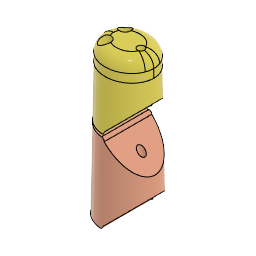
Thumb (Autodesk Fusion 360 design; units mm, degrees)
part number: 2025-12-08-00-09-45-361
part number: 2025-12-08-00-10-08-646
part number: 2025-12-08-00-15-25-462
Autodesk Fusion 360 part; units mm, degrees
sketch "Sketch1" plane through (0, 0, 0) normal (0, 0, 1) x (1, 0, 0) in component "Proximal phalanx"
  ellipse E0 centre (0, 0) end of major axis (0, -9) minor radius 10
  line L0 (0, 9) -> (0, -9) construction
  line L1 (-10, 0) -> (10, 0) construction
  dimension "d1" = 18
  dimension "d2" = 20
  constraint coincident E0 L0.start
  constraint coincident E0 L0.end
  constraint coincident E0 L1.start
  constraint coincident E0 L1.end
  constraint coincident E0.centre origin
  constraint vertical L0
  measures "d1" distance of E0
ref_plane "WorkPlane1" through (0, 0, 28) normal (0, 0, 1) x (1, 0, 0) in component "Proximal phalanx"
sketch "Sketch2" plane through (0, 0, 28) normal (0, 0, 1) x (1, 0, 0) in component "Proximal phalanx"
  ellipse E0 centre (0, 0) end of major axis (10, 0) minor radius 9
  spline S0 degree 3 poles (-9.5, 0) (-9.5, -2.2108) (-8.491, -4.4133) (-6.7366, -5.9923) (-5.0094, -7.5468) (-2.5777, -8.4723) (-0.1165, -8.4994) (2.3291, -8.5262) (4.7706, -7.6659) (6.5373, -6.1665) (8.3249, -4.6493) (9.4028, -2.5017) (9.4935, -0.3149) (9.5862, 1.9206) (8.6455, 4.1803) (6.9214, 5.8213) (5.2517, 7.4105) (2.8652, 8.3954) (0.4176, 8.4918) (-2.0105, 8.5874) (-4.4666, 7.8077) (-6.2824, 6.3751) (-8.121, 4.9244) (-9.2833, 2.8271) (-9.4715, 0.6572) (-9.4905, 0.4386) (-9.5, 0.2193) (-9.5, 0) knots -3.141593 -3.141593 -3.141593 -3.141593 -2.356194 -2.356194 -2.356194 -1.582994 -1.582994 -1.582994 -0.814704 -0.814704 -0.814704 -0.037301 -0.037301 -0.037301 0.757422 0.757422 0.757422 1.527054 1.527054 1.527054 2.290564 2.290564 2.290564 3.06369 3.06369 3.06369 3.141593 3.141593 3.141593 3.141593
  dimension "d4" = -0.5
loft "Loft1" add profiles "Sketch2", "Sketch1" section 1 contours S0 section 2 makes body 1 in component "Proximal phalanx"
sketch "Sketch3" plane through (0, 0, 28) normal (0, 0, 1) x (-1, 0, 0) in component "Proximal phalanx"
  spline S0 degree 3 poles (9.5, 0) (9.5, 2.2108) (8.491, 4.4133) (6.7366, 5.9923) (5.0094, 7.5468) (2.5777, 8.4723) (0.1165, 8.4994) (-2.3291, 8.5262) (-4.7706, 7.6659) (-6.5373, 6.1665) (-8.3249, 4.6493) (-9.4028, 2.5017) (-9.4935, 0.3149) (-9.5862, -1.9206) (-8.6455, -4.1803) (-6.9214, -5.8213) (-5.2517, -7.4105) (-2.8652, -8.3954) (-0.4176, -8.4918) (2.0105, -8.5874) (4.4666, -7.8077) (6.2824, -6.3751) (8.121, -4.9244) (9.2833, -2.8271) (9.4715, -0.6572) (9.4905, -0.4386) (9.5, -0.2193) (9.5, 0) knots -3.141593 -3.141593 -3.141593 -3.141593 -2.356194 -2.356194 -2.356194 -1.582994 -1.582994 -1.582994 -0.814704 -0.814704 -0.814704 -0.037301 -0.037301 -0.037301 0.757422 0.757422 0.757422 1.527054 1.527054 1.527054 2.290564 2.290564 2.290564 3.06369 3.06369 3.06369 3.141593 3.141593 3.141593 3.141593
  line L0 (0, 0) -> (-9.5, 0) construction
  circle A0 centre (-4.75, 0) radius 1.25
  dimension "d5" = 2.5
  constraint coincident L0.start origin
  constraint coincident S0 L0.end
  constraint horizontal L0
  constraint midpoint L0 A0.centre
  measures "d5" diameter of A0
extrude "Extrude1" cut sketch "Sketch3" against normal blind 33 contours A0 bodies 1 in component "Proximal phalanx"
ref_plane "WorkPlane2" through (0, 0, 0) normal (0, 1, 0) x (0, 0, 1) in component "Proximal phalanx"
sketch "Sketch4" plane through (0, 0, 0) normal (0, 1, 0) x (1, 0, 0) in component "Proximal phalanx"
  line L0 (0, -28) -> (0, -27)
  line L1 (0, -27) -> (10.3762, -16.6238)
  line L2 (10.3762, -16.6238) -> (10.3762, -28)
  line L3 (10.3762, -28) -> (0, -28)
  line L4 (0, 0) -> (0, -1)
  line L5 (0, -1) -> (10.59, -11.59)
  line L6 (10.59, -11.59) -> (10.59, 0)
  line L7 (10.59, 0) -> (0, 0)
  dimension "d9" = 1
  dimension "d10" = 45
  dimension "d11" = 1
  dimension "d12" = 45
  constraint vertical L0
  constraint parallel L0 L2
  constraint perpendicular L0 L3
  constraint coincident L4.start L7.end
  constraint vertical L4
  constraint parallel L4 L6
  constraint perpendicular L4 L7
  measures "d9" distance of L0.start L0.end
  measures "d10" angle of L1 L3
  measures "d11" distance of L4.start L4.end
  measures "d12" angle of L5 L7
extrude "Extrude2" cut sketch "Sketch4" along normal mid plane 20 bodies 1 in component "Proximal phalanx"
fillet "Fillet1" radius 1 2 edges at (0, 0, 28) (0, 0, 0) on bodies 1 in component "Proximal phalanx"
sketch "Sketch5" plane through (0, 0, 28) normal (0, 0, 1) x (-1, 0, 0) in component "Proximal phalanx"
  line L0 (1, 8.4527) -> (1, -8.4527)
  spline S0 degree 3 poles (1, -8.4527) (2.9442, -8.2685) (4.8202, -7.5288) (6.2824, -6.3751) (8.121, -4.9244) (9.2833, -2.8271) (9.4715, -0.6572) (9.4905, -0.4386) (9.5, -0.2193) (9.5, 0) knots 1.675706 1.675706 1.675706 1.675706 2.290564 2.290564 2.290564 3.06369 3.06369 3.06369 3.141593 3.141593 3.141593 3.141593
  spline S1 degree 3 poles (9.5, 0) (9.5, 2.2108) (8.491, 4.4133) (6.7366, 5.9923) (5.2165, 7.3604) (3.1519, 8.2488) (1, 8.4527) knots -3.141593 -3.141593 -3.141593 -3.141593 -2.356194 -2.356194 -2.356194 -1.675706 -1.675706 -1.675706 -1.675706
  line L1 (1, 0) -> (9.5, 0) construction
  line L2 (5.25, 0) -> (5.25, -7.0834) construction
  line L3 (5.25, -7.0834) -> (5.25, 0) construction
  line L4 (5.25, 0) -> (5.25, 7.0834) construction
  circle A0 centre (5.25, -3.5417) radius 2
  circle A1 centre (5.25, 3.5417) radius 2
  dimension "d17" = 4
  dimension "d18" = 4
  constraint midpoint L0 L1.start
  constraint coincident S0.end S1.start
  constraint midpoint L1 L2.start
  constraint coincident S0 L2.end
  constraint perpendicular L1 L2
  constraint coincident S1 L4.end
  constraint perpendicular L1 L4
  constraint midpoint L3 A0.centre
  constraint midpoint L4 A1.centre
  measures "d17" diameter of A0
  measures "d18" diameter of A1
extrude "Extrude3" cut sketch "Sketch5" against normal blind 41 contours A0 | A1 bodies 1 in component "Proximal phalanx"
ref_plane "WorkPlane1" through (-5.25, 0, 29) normal (0, 0, 1) x (1, 0, 0) in component "Distal phalanx"
sketch "Sketch1 (2)" plane through (0, 0, 29) normal (0, 0, 1) x (1, 0, 0) in component "Distal phalanx"
  spline S0 degree 3 poles (-9.5, 0) (-9.5, -2.2108) (-8.491, -4.4133) (-6.7366, -5.9923) (-5.0094, -7.5468) (-2.5777, -8.4723) (-0.1165, -8.4994) (2.3291, -8.5262) (4.7706, -7.6659) (6.5373, -6.1665) (8.3249, -4.6493) (9.4028, -2.5017) (9.4935, -0.3149) (9.5862, 1.9206) (8.6455, 4.1803) (6.9214, 5.8213) (5.2517, 7.4105) (2.8652, 8.3954) (0.4176, 8.4918) (-2.0105, 8.5874) (-4.4666, 7.8077) (-6.2824, 6.3751) (-8.121, 4.9244) (-9.2833, 2.8271) (-9.4715, 0.6572) (-9.4905, 0.4386) (-9.5, 0.2193) (-9.5, 0) knots -3.141593 -3.141593 -3.141593 -3.141593 -2.356194 -2.356194 -2.356194 -1.582994 -1.582994 -1.582994 -0.814704 -0.814704 -0.814704 -0.037301 -0.037301 -0.037301 0.757422 0.757422 0.757422 1.527054 1.527054 1.527054 2.290564 2.290564 2.290564 3.06369 3.06369 3.06369 3.141593 3.141593 3.141593 3.141593
ref_plane "WorkPlane2" through (0.0431, 0.0306, 47) normal (0, 0, 1) x (1, 0, 0) in component "Distal phalanx"
sketch "Sketch2 (2)" plane through (0, 0, 47) normal (0, 0, 1) x (1, 0, 0) in component "Distal phalanx"
  spline S0 degree 3 poles (-9.5, 0) (-9.5, -2.2108) (-8.491, -4.4133) (-6.7366, -5.9923) (-5.0094, -7.5468) (-2.5777, -8.4723) (-0.1165, -8.4994) (2.3291, -8.5262) (4.7706, -7.6659) (6.5373, -6.1665) (8.3249, -4.6493) (9.4028, -2.5017) (9.4935, -0.3149) (9.5862, 1.9206) (8.6455, 4.1803) (6.9214, 5.8213) (5.2517, 7.4105) (2.8652, 8.3954) (0.4176, 8.4918) (-2.0105, 8.5874) (-4.4666, 7.8077) (-6.2824, 6.3751) (-8.121, 4.9244) (-9.2833, 2.8271) (-9.4715, 0.6572) (-9.4905, 0.4386) (-9.5, 0.2193) (-9.5, 0) knots -3.141593 -3.141593 -3.141593 -3.141593 -2.356194 -2.356194 -2.356194 -1.582994 -1.582994 -1.582994 -0.814704 -0.814704 -0.814704 -0.037301 -0.037301 -0.037301 0.757422 0.757422 0.757422 1.527054 1.527054 1.527054 2.290564 2.290564 2.290564 3.06369 3.06369 3.06369 3.141593 3.141593 3.141593 3.141593
  spline S1 degree 3 poles (-9.2, 0) (-9.2, -2.1235) (-8.2323, -4.2426) (-6.5359, -5.7693) (-4.8678, -7.2707) (-2.5101, -8.1712) (-0.1213, -8.1993) (2.2306, -8.227) (4.5789, -7.4095) (6.2844, -5.9872) (8.0574, -4.5087) (9.1168, -2.4035) (9.1951, -0.2674) (9.2737, 1.8772) (8.3641, 4.0441) (6.6941, 5.6234) (5.072, 7.1573) (2.7469, 8.1093) (0.3646, 8.1936) (-1.9937, 8.277) (-4.3747, 7.5092) (-6.1241, 6.1178) (-7.931, 4.6807) (-9.045, 2.6049) (-9.1844, 0.4775) (-9.1948, 0.3185) (-9.2, 0.1592) (-9.2, 0) knots -3.141593 -3.141593 -3.141593 -3.141593 -2.356194 -2.356194 -2.356194 -1.583873 -1.583873 -1.583873 -0.82348 -0.82348 -0.82348 -0.032974 -0.032974 -0.032974 0.760668 0.760668 0.760668 1.5315 1.5315 1.5315 2.294553 2.294553 2.294553 3.082697 3.082697 3.082697 3.141593 3.141593 3.141593 3.141593
  dimension "d23" = -0.3
loft "Loft1'" add profiles "Sketch2 (2)", "Sketch1 (2)" section 1 contours S1 section 2 separate body makes body 2 in component "Distal phalanx"
sketch "Sketch3 (2)" plane through (0, 0, 47) normal (0, 0, 1) x (-1, 0, 0) in component "Distal phalanx"
  spline S0 degree 3 poles (9.2, 0) (9.2, 2.1235) (8.2323, 4.2426) (6.5359, 5.7693) (4.8678, 7.2707) (2.5101, 8.1712) (0.1213, 8.1993) (-2.2306, 8.227) (-4.5789, 7.4095) (-6.2844, 5.9872) (-8.0574, 4.5087) (-9.1168, 2.4035) (-9.1951, 0.2674) (-9.2737, -1.8772) (-8.3641, -4.0441) (-6.6941, -5.6234) (-5.072, -7.1573) (-2.7469, -8.1093) (-0.3646, -8.1936) (1.9937, -8.277) (4.3747, -7.5092) (6.1241, -6.1178) (7.931, -4.6807) (9.045, -2.6049) (9.1844, -0.4775) (9.1948, -0.3185) (9.2, -0.1592) (9.2, 0) knots -3.141593 -3.141593 -3.141593 -3.141593 -2.356194 -2.356194 -2.356194 -1.583873 -1.583873 -1.583873 -0.82348 -0.82348 -0.82348 -0.032974 -0.032974 -0.032974 0.760668 0.760668 0.760668 1.5315 1.5315 1.5315 2.294553 2.294553 2.294553 3.082697 3.082697 3.082697 3.141593 3.141593 3.141593 3.141593
  line L0 (0, 0) -> (-9.2, 0) construction
  circle A0 centre (-4.6, 0) radius 1.25
  dimension "d24" = 2.5
  constraint coincident L0.start origin
  constraint coincident S0 L0.end
  constraint horizontal L0
  constraint midpoint L0 A0.centre
  measures "d24" diameter of A0
extrude "Extrude1'" cut sketch "Sketch3 (2)" against normal blind 18 contours A0 bodies 2 in component "Distal phalanx"
ref_plane "WorkPlane3" through (0, 0, 0) normal (0, 1, 0) x (0, 0, 1) in component "Distal phalanx"
sketch "Sketch4 (2)" plane through (0, 0, 0) normal (0, 1, 0) x (1, 0, 0) in component "Distal phalanx"
  line L0 (0, -29) -> (0, -30)
  line L1 (0, -30) -> (10, -40)
  line L2 (10, -40) -> (10, -29)
  line L3 (10, -29) -> (0, -29)
  dimension "d28" = 45
  dimension "d29" = 1
  constraint vertical L0
  constraint parallel L0 L2
  constraint perpendicular L0 L3
  measures "d28" angle of L1 L3
  measures "d29" distance of L0.start L0.end
extrude "Extrude2'" cut sketch "Sketch4 (2)" along normal mid plane 20 bodies 2 in component "Distal phalanx"
sketch "Sketch5 (2)" plane through (0, 0, 47) normal (0, 0, 1) x (-1, 0, 0) in component "Distal phalanx"
  circle A0 centre (-4.6, 0) radius 1.25
  spline S0 degree 3 poles (9.2, 0) (9.2, 2.1235) (8.2323, 4.2426) (6.5359, 5.7693) (4.8678, 7.2707) (2.5101, 8.1712) (0.1213, 8.1993) (-2.2306, 8.227) (-4.5789, 7.4095) (-6.2844, 5.9872) (-8.0574, 4.5087) (-9.1168, 2.4035) (-9.1951, 0.2674) (-9.2737, -1.8772) (-8.3641, -4.0441) (-6.6941, -5.6234) (-5.072, -7.1573) (-2.7469, -8.1093) (-0.3646, -8.1936) (1.9937, -8.277) (4.3747, -7.5092) (6.1241, -6.1178) (7.931, -4.6807) (9.045, -2.6049) (9.1844, -0.4775) (9.1948, -0.3185) (9.2, -0.1592) (9.2, 0) knots -3.141593 -3.141593 -3.141593 -3.141593 -2.356194 -2.356194 -2.356194 -1.583873 -1.583873 -1.583873 -0.82348 -0.82348 -0.82348 -0.032974 -0.032974 -0.032974 0.760668 0.760668 0.760668 1.5315 1.5315 1.5315 2.294553 2.294553 2.294553 3.082697 3.082697 3.082697 3.141593 3.141593 3.141593 3.141593
  line L0 (0, 0) -> (9.2, 0) construction
  line L1 (4.6, 0) -> (4.6, 7.1004) construction
  line L2 (4.6, 0) -> (4.6, -7.1004) construction
  circle A1 centre (4.6, -3.5502) radius 2
  circle A2 centre (4.6, 3.5502) radius 2
  dimension "d32" = 4
  dimension "d33" = 4
  constraint coincident L0.start origin
  constraint coincident S0.start S0.end
  constraint midpoint L0 L1.start
  constraint coincident S0 L1.end
  constraint perpendicular L0 L1
  constraint coincident S0 L2.end
  constraint perpendicular L0 L2
  constraint midpoint L2 A1.centre
  constraint midpoint L1 A2.centre
  measures "d32" diameter of A1
  measures "d33" diameter of A2
extrude "Extrude3'" cut sketch "Sketch5 (2)" against normal blind 18 contours A1 | A2 bodies 2 in component "Distal phalanx"
extrude "Extrude4" add 1 faces at (1.2069, -4.2429, 47) along direction (0, 0, 1) blind 7 on bodies 2 bodies 2 in component "Distal phalanx"
fillet "Fillet1'" radius 4 1 edges at (9.1998, 0, 54) on bodies 2 in component "Distal phalanx"
fillet "Fillet2" radius 1 1 edges at (0, 0, 29) on bodies 2 in component "Distal phalanx"
component "Proximal phalanx" placed x (1, 0, 0) y (0, 1, 0) z (0, 0, 1) at (0, 0, 0)
component "Distal phalanx" placed x (1, 0, 0) y (0, 1, 0) z (0, 0, 1) at (0, 0, 0)
equation "d3 = 4.3 cm - 1.5 cm"
